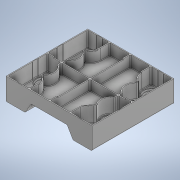
# Autodesk Inventor part: WarSunTray
Saved by Autodesk Inventor 2021 (Build 250183000, 183)
## iProperties
Created: 2023-03-17
Part Number: WarSunTray
Material: ABS Plastic
Document SubType Name: Modeling
Designer: Bradley
Density: 1.06 g/cm^3
Appearance: Smooth - Medium Gray
Author: Bradley
Autodesk Inventor part; units mm, degrees
ref_plane "YZ Plane" through (0, 0, 0) normal (1, 0, 0) x (0, 1, 0)
ref_plane "XZ Plane" through (0, 0, 0) normal (0, 1, 0) x (-1, 0, 0)
ref_plane "XY Plane" through (0, 0, 0) normal (0, 0, 1) x (1, 0, 0)
sketch "Sketch1" plane through (0, 0, 0) normal (0, 0, 1) x (1, 0, 0)
  line L0 (-75, 20.1) -> (-75, -17.9)
  line L1 (-75, -17.9) -> (-41.627, -17.9)
  line L2 (-41.627, -17.9) -> (-31.2924, 0)
  line L3 (-31.2924, 0) -> (31.2924, 0)
  line L4 (31.2924, 0) -> (41.627, -17.9)
  line L5 (41.627, -17.9) -> (75, -17.9)
  line L6 (75, -17.9) -> (75, 20.1)
  line L7 (-75, 20.1) -> (75, 20.1)
  line L8 (-31.2924, -0.5) -> (31.2924, -0.5) construction
  line L9 (31.2924, -0.5) -> (62.5848, -54.7) construction
  line L10 (62.5848, -54.7) -> (31.2924, -108.9) construction
  line L11 (31.2924, -108.9) -> (-31.2924, -108.9) construction
  line L12 (-31.2924, -108.9) -> (-62.5848, -54.7) construction
  line L13 (-62.5848, -54.7) -> (-31.2924, -0.5) construction
  line L14 (-75, -13.9) -> (-40.4723, -13.9)
  line L15 (-40.4723, -13.9) -> (-20.8423, 20.1)
  point P0 (0, 0)
  point P1 (0, 0)
  point P2 (0, 20.1)
  point P3 (0, -54.7)
  dimension "d0" = 75
  dimension "d2" = 38
  dimension "d3" = 108.4
  dimension "d4" = 0.5
  dimension "d5" = 0.25
  dimension "d6" = 91
  dimension "d53" = 20.1
  dimension "d115" = 4
  dimension "d116" = 1
  constraints: 32 end point, 4 point on line, 3 parallel, 3 perpendicular, 2 horizontal, 2 midpoint, 2 vertical alignment, 1 coincident, 1 collinear, 1 vertical, 13 other
  measures "d0" distance from line of point (0, 0) L0
  measures "d2" distance of L0.start L0.end
  measures "d3" distance between parallel lines of L11 L8
  measures "d4" distance between parallel lines of L8 L3
  measures "d5" distance between parallel lines of L13 L2
  measures "d6" distance between parallel lines of L11 L1
  measures "d53" distance between parallel lines of L3 L7
  measures "d115" distance between parallel lines of L1 L14
  measures "d116" distance between parallel lines of L2 L15
extrude "Extrusion1" add sketch "Sketch1" along normal mid plane 142.25
fillet "Fillet1" radius 2 6 edges at (-31.2924, 0, 0) (31.2924, 0, 0) (41.627, -17.9, 0) (-41.627, -17.9, 0) (-75, -17.9, 0) (75, -17.9, 0)
sketch "Sketch2" plane through (-75, 20.1, 71.125) normal (0, 1, 0) x (1, 0, 0)
  line L0 (0, 142.25) -> (0, 0) projected
  line L1 (150, 0) -> (0, 0) projected
  line L2 (150, 142.25) -> (150, 0) projected
  line L3 (0, 142.25) -> (150, 142.25) projected
  circle A0 centre (21.9, 124.95) radius 16 construction
  circle A1 centre (21.9, 124.95) radius 16.5 construction
  circle A2 centre (21.9, 124.95) radius 11.5 construction
  circle A3 centre (21.9, 124.95) radius 12
  circle A4 centre (21.9, 124.95) radius 17.3 construction
  line L4 (0, 142.25) -> (150, 142.25) construction
  line L5 (150, 142.25) -> (150, 0) construction
  line L6 (150, 0) -> (0, 0) construction
  line L7 (0, 142.25) -> (0, 0) construction
  line L8 (21.9, 124.95) -> (21.9, 141.45) construction
  line L9 (3.6, 140.65) -> (36.4, 140.65)
  line L10 (38.4, 138.65) -> (38.4, 124.95)
  line L11 (25, 71.925) -> (3.6, 71.925)
  line L12 (1.6, 73.925) -> (1.6, 138.65)
  arc A5 (3.6, 140.65) -> (1.6, 138.65) centre (3.6, 138.65) ccw
  arc A6 (38.4, 138.65) -> (36.4, 140.65) centre (36.4, 138.65) ccw
  arc A7 (1.6, 73.925) -> (3.6, 71.925) centre (3.6, 73.925) ccw
  line L13 (33.9504, 142.25) -> (33.9504, 0) projected
  line L14 (32.2183, 0) -> (32.2183, 142.25) projected
  circle A8 centre (17.3, 92.7772) radius 17.3 construction
  circle A9 centre (17.3, 92.7772) radius 16.5 construction
  circle A10 centre (17.3, 92.7772) radius 16 construction
  circle A11 centre (17.3, 92.7772) radius 12
  line L15 (28.091, 36.4858) -> (21.547, 94.4298) construction
  line L16 (21.547, 94.4298) -> (68.4561, 129.069) construction
  line L17 (68.4561, 129.069) -> (121.909, 105.7642) construction
  line L18 (121.909, 105.7642) -> (128.453, 47.8202) construction
  line L19 (128.453, 47.8202) -> (81.5439, 13.181) construction
  line L20 (81.5439, 13.181) -> (28.091, 36.4858) construction
  arc A12 (9.6365, 92.4062) -> (27.5325, 41.4308) centre (106.7579, 97.8737) ccw construction
  arc A13 (9.6365, 92.4062) -> (22.41, 86.7886) centre (25.4971, 111.1395) ccw construction
  circle A14 centre (21.9, 124.95) radius 4 construction
  circle A15 centre (17.3, 92.7772) radius 4 construction
  circle A16 centre (17.3, 49.4728) radius 4 construction
  line L21 (17.3, 92.7772) -> (17.3, 49.4728) construction
  circle A17 centre (17.3, 92.7772) radius 4.437 construction
  circle A18 centre (17.3, 49.4728) radius 4.437 construction
  arc A19 (26.9754, 140.65) -> (16.8246, 140.65) centre (21.9, 124.95) ccw
  arc A20 (1.6, 97.8526) -> (1.6, 87.7018) centre (17.3, 92.7772) ccw
  line L22 (75, 71.125) -> (27.6265, 36.1428)
  line L23 (27.6265, 36.1428) -> (21.0178, 94.6606)
  line L24 (21.0178, 94.6606) -> (75, 71.125)
  arc A21 (9.0773, 93.5727) -> (27.0501, 41.2463) centre (106.7579, 97.8737) ccw
  arc A22 (9.0773, 93.5727) -> (21.8408, 87.3733) centre (25.4971, 111.1395) ccw
  line L25 (25, 71.925) -> (25, 78.184)
  arc A23 (25, 78.184) -> (27.262, 105.9305) centre (17.3, 92.7772) ccw
  arc A24 (27.7769, 109.5321) -> (38.4, 124.95) centre (21.9, 124.95) ccw
  line L26 (21.9, 124.95) -> (17.3, 92.7772) construction
  line L27 (27.7769, 109.5321) -> (27.262, 105.9305)
  point P0 (17.3, 71.125)
  dimension "d10" = 32
  dimension "d13" = 23
  dimension "d23" = 0.8
  dimension "d26" = 24
  dimension "d27" = 33
  dimension "d28" = 2
  dimension "d70" = 4.9765
  dimension "d71" = 7.6898
  dimension "d72" = 101
  dimension "d73" = 97.2752
  dimension "d74" = 24.5458
  dimension "d75" = 8
  dimension "d76" = 12.0624
  dimension "d77" = 5.4473
  dimension "d78" = 1.6
  dimension "d79" = 1.6
  dimension "d80" = 0.8
  dimension "d81" = 21.9
  dimension "d84" = 0.5
  dimension "d85" = 0.5
  dimension "d86" = 0.5
  dimension "d106" = 25
  dimension "d107" = 8
  constraints: 36 end point, 31 point on circle, 25 centre point, 12 coincident, 12 tangent, 11 equal radius, 10 point on line, 4 concentric, 4 parallel, 3 vertical, 1 horizontal, 1 horizontal alignment, 1 midpoint, 1 perpendicular, 1 vertical alignment, 13 other
  measures "d10" diameter of A0
  measures "d13" diameter of A2
  measures "d23" radial gap between concentric circles of A1 A4
  measures "d26" diameter of A3
  measures "d27" diameter of A1
  measures "d28" radius of A5
  measures "d70" distance of L15.start A12.end
  measures "d71" distance of A13.end L15.end
  measures "d72" distance between parallel lines of L18 L15
  measures "d73" radius of A12
  measures "d74" radius of A13
  measures "d75" diameter of A14
  measures "d76" distance from line of A12.start L15
  measures "d77" distance from line of A12.start L16
  measures "d78" distance between parallel lines of L9 L3
  measures "d79" distance between parallel lines of L12 L0
  measures "d80" distance from line of L11 point (17.3, 71.125)
  measures "d81" distance from line of A0.centre L0
  measures "d84" distance between parallel lines of L15 L23
  measures "d85" radial gap between concentric circles of A12 A21
  measures "d86" radial gap between concentric circles of A13 A22
  measures "d106" distance between parallel lines of L0 L25
  measures "d107" distance between parallel lines of L27 L26
extrude "Extrusion2" cut sketch "Sketch2" against normal blind 37 contours L14 A3 | A3 L14 | L24 L23 A22 A21 A11 | A11 L23 L24 | A11 A21 A22 L23
extrude "Extrusion3" cut sketch "Sketch2" against normal blind 27 contours L14 A3 A24 L27 A23 L24 A11 A21 L11 A7 L12 A5 L9 | L9 L13 A24 L14 A3 | L9 A6 L10 A24 L13 | L9 A19 | L14 A3 | A3 L14 | A23 L25 L11 L23 A11 L24 L14 | L14 L24 A23 | L14 A23 L24 | L24 L23 A22 A21 A11 | A11 L23 L24 | L11 A21 A11 L23 | A11 A21 A22 L23 | L12 A20
chamfer "Chamfer1" distance 2 angle 45 2 edges at (-65.1, -6.9, -53.825) (-69.7, -6.9, -21.6522)
fillet "Fillet3" radius 1 20 edges at (-65.1, -16.9, -53.825) (-65.1, -8.9, -53.825) (-67.1, -6.9, -53.825) (-53.1, -6.9, -70.325) (-72.8142, -6.9, -68.9392) (-73.4, -6.9, -47.1263) (-64.7877, -6.9, -69.525) (-37.1858, -6.9, -68.9392) (-36.6, -6.9, -60.675) (-60.7, -6.9, -0.8) (-72.8142, -6.9, -1.3858) (-73.4, -6.9, -9.6884) (-43.3123, -6.9, -69.525) (-74.2, -6.9, -21.6522) (-71.7, -6.9, -21.6522) (-69.7, -8.9, -21.6522) (-69.7, -16.9, -21.6522) (-47.4805, -6.9, -36.6063) (-41.2546, -6.9, -20.3115) (-50, -6.9, -3.9295)
fillet "Fillet3" radius 5 4 edges at (-73.4, 6.6, -26.7276) (-73.4, 6.6, -16.5768) (-58.1754, 6.6, -69.525) (-48.0246, 6.6, -69.525)
fillet "Fillet3" radius 2 1 edges at (-50, 6.6, -0.8)
fillet "Fillet3" radius 3 3 edges at (-47.738, 6.6, -34.8055) (-47.2231, 6.6, -38.4071) (-50, 6.6, -7.059)
sketch "Sketch6" plane through (-75, 20.1, 71.125) normal (0, 1, 0) x (1, 0, 0)
  arc A0 (26.3538, 78.9831) -> (25, 76.475) centre (28, 76.475) ccw projected
  line L0 (25, 76.475) -> (25, 73.925) projected
  arc A1 (23, 71.925) -> (25, 73.925) centre (23, 73.925) ccw projected
  line L1 (23, 71.925) -> (3.6, 71.925) projected
  arc A2 (1.6, 73.925) -> (3.6, 71.925) centre (3.6, 73.925) ccw projected
  line L2 (1.6, 73.925) -> (1.6, 86.9668) projected
  arc A3 (1.6, 86.9668) -> (1.414, 88.3181) centre (-3.4, 86.9668) ccw projected
  arc A4 (1.414, 97.2363) -> (1.414, 88.3181) centre (17.3, 92.7772) ccw projected
  arc A5 (1.414, 97.2363) -> (1.6, 98.5875) centre (-3.4, 98.5875) ccw projected
  line L3 (1.6, 98.5875) -> (1.6, 138.65) projected
  arc A6 (3.6, 140.65) -> (1.6, 138.65) centre (3.6, 138.65) ccw projected
  line L4 (3.6, 140.65) -> (16.0897, 140.65) projected
  arc A7 (16.0897, 140.65) -> (17.4409, 140.836) centre (16.0897, 145.65) ccw projected
  arc A8 (26.3591, 140.836) -> (17.4409, 140.836) centre (21.9, 124.95) ccw projected
  arc A9 (26.3591, 140.836) -> (27.7103, 140.65) centre (27.7103, 145.65) ccw projected
  line L5 (27.7103, 140.65) -> (36.4, 140.65) projected
  arc A10 (38.4, 138.65) -> (36.4, 140.65) centre (36.4, 138.65) ccw projected
  line L6 (38.4, 138.65) -> (38.4, 124.95) projected
  arc A11 (29.1857, 110.1456) -> (38.4, 124.95) centre (21.9, 124.95) ccw projected
  arc A12 (29.1857, 110.1456) -> (27.5405, 107.8785) centre (30.5103, 107.4539) ccw projected
  line L7 (27.5405, 107.8785) -> (27.4984, 107.584) projected
  arc A13 (27.4984, 107.584) -> (28.4423, 104.9468) centre (30.4682, 107.1594) ccw projected
  arc A14 (26.3538, 78.9831) -> (28.4423, 104.9468) centre (17.3, 92.7772) ccw projected
  line L8 (0, 142.25) -> (0, 0) projected
  line L9 (150, 0) -> (0, 0) projected
  line L10 (150, 142.25) -> (150, 0) projected
  line L11 (0, 142.25) -> (150, 142.25) projected
  line L12 (40, 124.95) -> (40, 138.65)
  arc A15 (40, 138.65) -> (36.4, 142.25) centre (36.4, 138.65) ccw
  line L13 (36.4, 142.25) -> (27.7103, 142.25)
  arc A16 (26.7915, 142.3765) -> (27.7103, 142.25) centre (27.7103, 145.65) ccw
  arc A17 (26.7915, 142.3765) -> (17.0085, 142.3765) centre (21.9, 124.95) ccw
  arc A18 (16.0897, 142.25) -> (17.0085, 142.3765) centre (16.0897, 145.65) ccw
  line L14 (16.0897, 142.25) -> (3.6, 142.25)
  arc A19 (3.6, 142.25) -> (0, 138.65) centre (3.6, 138.65) ccw
  line L15 (0, 138.65) -> (0, 98.5875)
  arc A20 (-0.1265, 97.6687) -> (0, 98.5875) centre (-3.4, 98.5875) ccw
  arc A21 (-0.1265, 97.6687) -> (-0.1265, 87.8857) centre (17.3, 92.7772) ccw
  arc A22 (0, 86.9668) -> (-0.1265, 87.8857) centre (-3.4, 86.9668) ccw
  line L16 (0, 86.9668) -> (0, 73.925)
  arc A23 (0, 73.925) -> (3.6, 70.325) centre (3.6, 73.925) ccw
  line L17 (3.6, 70.325) -> (23, 70.325)
  arc A24 (23, 70.325) -> (26.6, 73.925) centre (23, 73.925) ccw
  line L18 (26.6, 73.925) -> (26.6, 76.475)
  arc A25 (27.2318, 77.6454) -> (26.6, 76.475) centre (28, 76.475) ccw
  arc A26 (27.2318, 77.6454) -> (29.5228, 106.1268) centre (17.3, 92.7772) ccw
  arc A27 (29.0823, 107.3576) -> (29.5228, 106.1268) centre (30.4682, 107.1594) ccw
  line L19 (29.0823, 107.3576) -> (29.1244, 107.6521)
  arc A28 (29.8921, 108.7101) -> (29.1244, 107.6521) centre (30.5103, 107.4539) ccw
  arc A29 (29.8921, 108.7101) -> (40, 124.95) centre (21.9, 124.95) ccw
  arc A30 (42, 140.65) -> (40, 138.65) centre (42, 138.65) ccw
  arc A31 (26.6, 73.925) -> (28.6, 71.925) centre (28.6, 73.925) ccw
  arc A32 (72.2, 71.925) -> (74.2, 73.925) centre (72.2, 73.925) ccw
  arc A33 (74.2, 138.65) -> (72.2, 140.65) centre (72.2, 138.65) ccw
  line L20 (42, 140.65) -> (72.2, 140.65)
  line L21 (74.2, 138.65) -> (74.2, 73.925)
  line L22 (72.2, 71.925) -> (28.6, 71.925)
  line L23 (44.8623, 142.25) -> (44.8623, 0) projected
  line L24 (39.7975, 122.25) -> (44.8623, 122.25)
  point P0 (75, 71.125)
  point P1 (44.8623, 71.925)
  point P2 (44.8623, 140.65)
  dimension "d110" = 0.8
  dimension "d121" = 20
  constraints: 39 point on circle, 24 end point, 19 centre point, 8 tangent, 3 collinear, 2 equal radius, 1 parallel, 1 perpendicular, 1 point on line, 1 vertical, 22 other
  measures "d110" distance from line of point (75, 71.125) L21
  measures "d121" distance between parallel lines of L24 L11
extrude "Extrusion8" cut sketch "Sketch6" against normal blind 19.1 contours A30 L20 L23 L24 A29 L12 | L20 A33 L21 A32 L22 L23 | L22 A31 L18 A25 A26 A27 L19 A28 A29 L24 L23
fillet "Fillet4" radius 1 8 edges at (-1.3858, 1, -1.3858) (-0.8, 1, -35.1625) (-1.3858, 1, -68.9392) (-17.9, 1, -69.525) (-34.4142, 1, -68.9392) (-35, 1, -60.675) (-37.7334, 1, -44.2607) (-24.6, 1, -0.8)
mirror "Mirror1" about plane through (0, 0, 0) normal (1, 0, 0) of "Extrusion2", "Extrusion3", "Chamfer1", "Fillet3", "Extrusion8", "Fillet4"
mirror "Mirror2" about plane through (0, 0, 0) normal (0, 0, 1) of "Extrusion2", "Extrusion3", "Chamfer1", "Fillet3", "Mirror1", "Extrusion8", "Fillet4"
extrude "Extrusion6" cut sketch "Sketch2" against normal blind 2 contours L22 L23 L11 L25 A23 L14 | L14 A23 L24 L13 L22 | L13 L24 L22 | A23 L25 L11 L23 A11 L24 L14 | L14 L24 A23 | A21 L11 L23 | A11 L23 L24 | L11 A21 A11 L23 | A11 A21 A22 L23 picked at (32.3812, 87.4589)
pattern_circular "Circular Pattern1" count 6 over 360 about axis through (0, -10, 0) along (0, 1, 0) of "Extrusion6"
equation "\"d2\" = Depth"
equation "\"d3\" = Outside"
equation "\"Depth\" = 38"
equation "\"Outside\" = 108.4"
body "Solid1"
